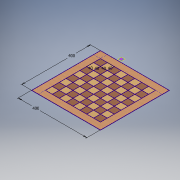
# Autodesk Inventor part: Lid
Saved by Autodesk Inventor 2019 (Build 230136000, 136)
## iProperties
Created: 2019-08-21
Part Number: Lid
Material: Generic
Document SubType Name: Modeling
Designer: Bruno
Density: 1 g/cm^3
Appearance: Default
Author: Bruno
Autodesk Inventor part; units mm, degrees
ref_plane "YZ Plane" through (0, 0, 0) normal (1, 0, 0) x (0, 1, 0)
ref_plane "XZ Plane" through (0, 0, 0) normal (0, 1, 0) x (-1, 0, 0)
ref_plane "XY Plane" through (0, 0, 0) normal (0, 0, 1) x (1, 0, 0)
ref_plane "Work Plane4" through (0, -2, 0) normal (0, -1, 0) x (1, 0, 0)
sketch "Sketch2" plane through (0, -2, 0) normal (0, -1, 0) x (1, 0, 0)
  line L0 (-64.9312, 57.9049) -> (-24.9312, 57.9049)
  line L1 (-24.9312, 57.9049) -> (-24.9312, 97.9049)
  line L2 (-24.9312, 97.9049) -> (-64.9312, 97.9049)
  line L3 (-64.9312, 97.9049) -> (-64.9312, 57.9049)
  line L4 (-24.9312, 137.9049) -> (-64.9312, 137.9049)
  line L5 (-24.9312, 97.9049) -> (-24.9312, 137.9049)
  line L6 (-64.9312, 97.9049) -> (-24.9312, 97.9049)
  line L7 (-64.9312, 137.9049) -> (-64.9312, 97.9049)
  line L8 (-24.9312, 177.9049) -> (-64.9312, 177.9049)
  line L9 (-24.9312, 137.9049) -> (-24.9312, 177.9049)
  line L10 (-64.9312, 137.9049) -> (-24.9312, 137.9049)
  line L11 (-64.9312, 177.9049) -> (-64.9312, 137.9049)
  line L12 (-24.9312, 217.9049) -> (-64.9312, 217.9049)
  line L13 (-24.9312, 177.9049) -> (-24.9312, 217.9049)
  line L14 (-64.9312, 177.9049) -> (-24.9312, 177.9049)
  line L15 (-64.9312, 217.9049) -> (-64.9312, 177.9049)
  line L16 (-24.9312, 257.9049) -> (-64.9312, 257.9049)
  line L17 (-24.9312, 217.9049) -> (-24.9312, 257.9049)
  line L18 (-64.9312, 217.9049) -> (-24.9312, 217.9049)
  line L19 (-64.9312, 257.9049) -> (-64.9312, 217.9049)
  line L20 (-24.9312, 297.9049) -> (-64.9312, 297.9049)
  line L21 (-24.9312, 257.9049) -> (-24.9312, 297.9049)
  line L22 (-64.9312, 257.9049) -> (-24.9312, 257.9049)
  line L23 (-64.9312, 297.9049) -> (-64.9312, 257.9049)
  line L24 (-24.9312, 337.9049) -> (-64.9312, 337.9049)
  line L25 (-24.9312, 297.9049) -> (-24.9312, 337.9049)
  line L26 (-64.9312, 297.9049) -> (-24.9312, 297.9049)
  line L27 (-64.9312, 337.9049) -> (-64.9312, 297.9049)
  line L28 (-24.9312, 377.9049) -> (-64.9312, 377.9049)
  line L29 (-24.9312, 337.9049) -> (-24.9312, 377.9049)
  line L30 (-64.9312, 337.9049) -> (-24.9312, 337.9049)
  line L31 (-64.9312, 377.9049) -> (-64.9312, 337.9049)
  line L32 (15.0688, 97.9049) -> (-24.9312, 97.9049)
  line L33 (15.0688, 57.9049) -> (15.0688, 97.9049)
  line L34 (-24.9312, 57.9049) -> (15.0688, 57.9049)
  line L35 (-24.9312, 97.9049) -> (-24.9312, 57.9049)
  line L36 (15.0688, 137.9049) -> (-24.9312, 137.9049)
  line L37 (15.0688, 97.9049) -> (15.0688, 137.9049)
  line L38 (-24.9312, 97.9049) -> (15.0688, 97.9049)
  line L39 (-24.9312, 137.9049) -> (-24.9312, 97.9049)
  line L40 (15.0688, 177.9049) -> (-24.9312, 177.9049)
  line L41 (15.0688, 137.9049) -> (15.0688, 177.9049)
  line L42 (-24.9312, 137.9049) -> (15.0688, 137.9049)
  line L43 (-24.9312, 177.9049) -> (-24.9312, 137.9049)
  line L44 (15.0688, 217.9049) -> (-24.9312, 217.9049)
  line L45 (15.0688, 177.9049) -> (15.0688, 217.9049)
  line L46 (-24.9312, 177.9049) -> (15.0688, 177.9049)
  line L47 (-24.9312, 217.9049) -> (-24.9312, 177.9049)
  line L48 (15.0688, 257.9049) -> (-24.9312, 257.9049)
  line L49 (15.0688, 217.9049) -> (15.0688, 257.9049)
  line L50 (-24.9312, 217.9049) -> (15.0688, 217.9049)
  line L51 (-24.9312, 257.9049) -> (-24.9312, 217.9049)
  line L52 (15.0688, 297.9049) -> (-24.9312, 297.9049)
  line L53 (15.0688, 257.9049) -> (15.0688, 297.9049)
  line L54 (-24.9312, 257.9049) -> (15.0688, 257.9049)
  line L55 (-24.9312, 297.9049) -> (-24.9312, 257.9049)
  line L56 (15.0688, 337.9049) -> (-24.9312, 337.9049)
  line L57 (15.0688, 297.9049) -> (15.0688, 337.9049)
  line L58 (-24.9312, 297.9049) -> (15.0688, 297.9049)
  line L59 (-24.9312, 337.9049) -> (-24.9312, 297.9049)
  line L60 (15.0688, 377.9049) -> (-24.9312, 377.9049)
  line L61 (15.0688, 337.9049) -> (15.0688, 377.9049)
  line L62 (-24.9312, 337.9049) -> (15.0688, 337.9049)
  line L63 (-24.9312, 377.9049) -> (-24.9312, 337.9049)
  line L64 (55.0688, 97.9049) -> (15.0688, 97.9049)
  line L65 (55.0688, 57.9049) -> (55.0688, 97.9049)
  line L66 (15.0688, 57.9049) -> (55.0688, 57.9049)
  line L67 (15.0688, 97.9049) -> (15.0688, 57.9049)
  line L68 (55.0688, 137.9049) -> (15.0688, 137.9049)
  line L69 (55.0688, 97.9049) -> (55.0688, 137.9049)
  line L70 (15.0688, 97.9049) -> (55.0688, 97.9049)
  line L71 (15.0688, 137.9049) -> (15.0688, 97.9049)
  line L72 (55.0688, 177.9049) -> (15.0688, 177.9049)
  line L73 (55.0688, 137.9049) -> (55.0688, 177.9049)
  line L74 (15.0688, 137.9049) -> (55.0688, 137.9049)
  line L75 (15.0688, 177.9049) -> (15.0688, 137.9049)
  line L76 (55.0688, 217.9049) -> (15.0688, 217.9049)
  line L77 (55.0688, 177.9049) -> (55.0688, 217.9049)
  line L78 (15.0688, 177.9049) -> (55.0688, 177.9049)
  line L79 (15.0688, 217.9049) -> (15.0688, 177.9049)
  line L80 (55.0688, 257.9049) -> (15.0688, 257.9049)
  line L81 (55.0688, 217.9049) -> (55.0688, 257.9049)
  line L82 (15.0688, 217.9049) -> (55.0688, 217.9049)
  line L83 (15.0688, 257.9049) -> (15.0688, 217.9049)
  line L84 (55.0688, 297.9049) -> (15.0688, 297.9049)
  line L85 (55.0688, 257.9049) -> (55.0688, 297.9049)
  line L86 (15.0688, 257.9049) -> (55.0688, 257.9049)
  line L87 (15.0688, 297.9049) -> (15.0688, 257.9049)
  line L88 (55.0688, 337.9049) -> (15.0688, 337.9049)
  line L89 (55.0688, 297.9049) -> (55.0688, 337.9049)
  line L90 (15.0688, 297.9049) -> (55.0688, 297.9049)
  line L91 (15.0688, 337.9049) -> (15.0688, 297.9049)
  line L92 (55.0688, 377.9049) -> (15.0688, 377.9049)
  line L93 (55.0688, 337.9049) -> (55.0688, 377.9049)
  line L94 (15.0688, 337.9049) -> (55.0688, 337.9049)
  line L95 (15.0688, 377.9049) -> (15.0688, 337.9049)
  line L96 (95.0688, 97.9049) -> (55.0688, 97.9049)
  line L97 (95.0688, 57.9049) -> (95.0688, 97.9049)
  line L98 (55.0688, 57.9049) -> (95.0688, 57.9049)
  line L99 (55.0688, 97.9049) -> (55.0688, 57.9049)
  line L100 (95.0688, 137.9049) -> (55.0688, 137.9049)
  line L101 (95.0688, 97.9049) -> (95.0688, 137.9049)
  line L102 (55.0688, 97.9049) -> (95.0688, 97.9049)
  line L103 (55.0688, 137.9049) -> (55.0688, 97.9049)
  line L104 (95.0688, 177.9049) -> (55.0688, 177.9049)
  line L105 (95.0688, 137.9049) -> (95.0688, 177.9049)
  line L106 (55.0688, 137.9049) -> (95.0688, 137.9049)
  line L107 (55.0688, 177.9049) -> (55.0688, 137.9049)
  line L108 (95.0688, 217.9049) -> (55.0688, 217.9049)
  line L109 (95.0688, 177.9049) -> (95.0688, 217.9049)
  line L110 (55.0688, 177.9049) -> (95.0688, 177.9049)
  line L111 (55.0688, 217.9049) -> (55.0688, 177.9049)
  line L112 (95.0688, 257.9049) -> (55.0688, 257.9049)
  line L113 (95.0688, 217.9049) -> (95.0688, 257.9049)
  line L114 (55.0688, 217.9049) -> (95.0688, 217.9049)
  line L115 (55.0688, 257.9049) -> (55.0688, 217.9049)
  line L116 (95.0688, 297.9049) -> (55.0688, 297.9049)
  line L117 (95.0688, 257.9049) -> (95.0688, 297.9049)
  line L118 (55.0688, 257.9049) -> (95.0688, 257.9049)
  line L119 (55.0688, 297.9049) -> (55.0688, 257.9049)
  line L120 (95.0688, 337.9049) -> (55.0688, 337.9049)
  line L121 (95.0688, 297.9049) -> (95.0688, 337.9049)
  line L122 (55.0688, 297.9049) -> (95.0688, 297.9049)
  line L123 (55.0688, 337.9049) -> (55.0688, 297.9049)
  line L124 (95.0688, 377.9049) -> (55.0688, 377.9049)
  line L125 (95.0688, 337.9049) -> (95.0688, 377.9049)
  line L126 (55.0688, 337.9049) -> (95.0688, 337.9049)
  line L127 (55.0688, 377.9049) -> (55.0688, 337.9049)
  line L128 (135.0688, 97.9049) -> (95.0688, 97.9049)
  line L129 (135.0688, 57.9049) -> (135.0688, 97.9049)
  line L130 (95.0688, 57.9049) -> (135.0688, 57.9049)
  line L131 (95.0688, 97.9049) -> (95.0688, 57.9049)
  line L132 (135.0688, 137.9049) -> (95.0688, 137.9049)
  line L133 (135.0688, 97.9049) -> (135.0688, 137.9049)
  line L134 (95.0688, 97.9049) -> (135.0688, 97.9049)
  line L135 (95.0688, 137.9049) -> (95.0688, 97.9049)
  line L136 (135.0688, 177.9049) -> (95.0688, 177.9049)
  line L137 (135.0688, 137.9049) -> (135.0688, 177.9049)
  line L138 (95.0688, 137.9049) -> (135.0688, 137.9049)
  line L139 (95.0688, 177.9049) -> (95.0688, 137.9049)
  line L140 (135.0688, 217.9049) -> (95.0688, 217.9049)
  line L141 (135.0688, 177.9049) -> (135.0688, 217.9049)
  line L142 (95.0688, 177.9049) -> (135.0688, 177.9049)
  line L143 (95.0688, 217.9049) -> (95.0688, 177.9049)
  line L144 (135.0688, 257.9049) -> (95.0688, 257.9049)
  line L145 (135.0688, 217.9049) -> (135.0688, 257.9049)
  line L146 (95.0688, 217.9049) -> (135.0688, 217.9049)
  line L147 (95.0688, 257.9049) -> (95.0688, 217.9049)
  line L148 (135.0688, 297.9049) -> (95.0688, 297.9049)
  line L149 (135.0688, 257.9049) -> (135.0688, 297.9049)
  line L150 (95.0688, 257.9049) -> (135.0688, 257.9049)
  line L151 (95.0688, 297.9049) -> (95.0688, 257.9049)
  line L152 (135.0688, 337.9049) -> (95.0688, 337.9049)
  line L153 (135.0688, 297.9049) -> (135.0688, 337.9049)
  line L154 (95.0688, 297.9049) -> (135.0688, 297.9049)
  line L155 (95.0688, 337.9049) -> (95.0688, 297.9049)
  line L156 (135.0688, 377.9049) -> (95.0688, 377.9049)
  line L157 (135.0688, 337.9049) -> (135.0688, 377.9049)
  line L158 (95.0688, 337.9049) -> (135.0688, 337.9049)
  line L159 (95.0688, 377.9049) -> (95.0688, 337.9049)
  line L160 (175.0688, 97.9049) -> (135.0688, 97.9049)
  line L161 (175.0688, 57.9049) -> (175.0688, 97.9049)
  line L162 (135.0688, 57.9049) -> (175.0688, 57.9049)
  line L163 (135.0688, 97.9049) -> (135.0688, 57.9049)
  line L164 (175.0688, 137.9049) -> (135.0688, 137.9049)
  line L165 (175.0688, 97.9049) -> (175.0688, 137.9049)
  line L166 (135.0688, 97.9049) -> (175.0688, 97.9049)
  line L167 (135.0688, 137.9049) -> (135.0688, 97.9049)
  line L168 (175.0688, 177.9049) -> (135.0688, 177.9049)
  line L169 (175.0688, 137.9049) -> (175.0688, 177.9049)
  line L170 (135.0688, 137.9049) -> (175.0688, 137.9049)
  line L171 (135.0688, 177.9049) -> (135.0688, 137.9049)
  line L172 (175.0688, 217.9049) -> (135.0688, 217.9049)
  line L173 (175.0688, 177.9049) -> (175.0688, 217.9049)
  line L174 (135.0688, 177.9049) -> (175.0688, 177.9049)
  line L175 (135.0688, 217.9049) -> (135.0688, 177.9049)
  line L176 (175.0688, 257.9049) -> (135.0688, 257.9049)
  line L177 (175.0688, 217.9049) -> (175.0688, 257.9049)
  line L178 (135.0688, 217.9049) -> (175.0688, 217.9049)
  line L179 (135.0688, 257.9049) -> (135.0688, 217.9049)
  line L180 (175.0688, 297.9049) -> (135.0688, 297.9049)
  line L181 (175.0688, 257.9049) -> (175.0688, 297.9049)
  line L182 (135.0688, 257.9049) -> (175.0688, 257.9049)
  line L183 (135.0688, 297.9049) -> (135.0688, 257.9049)
  line L184 (175.0688, 337.9049) -> (135.0688, 337.9049)
  line L185 (175.0688, 297.9049) -> (175.0688, 337.9049)
  line L186 (135.0688, 297.9049) -> (175.0688, 297.9049)
  line L187 (135.0688, 337.9049) -> (135.0688, 297.9049)
  line L188 (175.0688, 377.9049) -> (135.0688, 377.9049)
  line L189 (175.0688, 337.9049) -> (175.0688, 377.9049)
  line L190 (135.0688, 337.9049) -> (175.0688, 337.9049)
  line L191 (135.0688, 377.9049) -> (135.0688, 337.9049)
  line L192 (215.0688, 97.9049) -> (175.0688, 97.9049)
  line L193 (215.0688, 57.9049) -> (215.0688, 97.9049)
  line L194 (175.0688, 57.9049) -> (215.0688, 57.9049)
  line L195 (175.0688, 97.9049) -> (175.0688, 57.9049)
  line L196 (215.0688, 137.9049) -> (175.0688, 137.9049)
  line L197 (215.0688, 97.9049) -> (215.0688, 137.9049)
  line L198 (175.0688, 97.9049) -> (215.0688, 97.9049)
  line L199 (175.0688, 137.9049) -> (175.0688, 97.9049)
  line L200 (215.0688, 177.9049) -> (175.0688, 177.9049)
  line L201 (215.0688, 137.9049) -> (215.0688, 177.9049)
  line L202 (175.0688, 137.9049) -> (215.0688, 137.9049)
  line L203 (175.0688, 177.9049) -> (175.0688, 137.9049)
  line L204 (215.0688, 217.9049) -> (175.0688, 217.9049)
  line L205 (215.0688, 177.9049) -> (215.0688, 217.9049)
  line L206 (175.0688, 177.9049) -> (215.0688, 177.9049)
  line L207 (175.0688, 217.9049) -> (175.0688, 177.9049)
  line L208 (215.0688, 257.9049) -> (175.0688, 257.9049)
  line L209 (215.0688, 217.9049) -> (215.0688, 257.9049)
  line L210 (175.0688, 217.9049) -> (215.0688, 217.9049)
  line L211 (175.0688, 257.9049) -> (175.0688, 217.9049)
  line L212 (215.0688, 297.9049) -> (175.0688, 297.9049)
  line L213 (215.0688, 257.9049) -> (215.0688, 297.9049)
  line L214 (175.0688, 257.9049) -> (215.0688, 257.9049)
  line L215 (175.0688, 297.9049) -> (175.0688, 257.9049)
  line L216 (215.0688, 337.9049) -> (175.0688, 337.9049)
  line L217 (215.0688, 297.9049) -> (215.0688, 337.9049)
  line L218 (175.0688, 297.9049) -> (215.0688, 297.9049)
  line L219 (175.0688, 337.9049) -> (175.0688, 297.9049)
  line L220 (215.0688, 377.9049) -> (175.0688, 377.9049)
  line L221 (215.0688, 337.9049) -> (215.0688, 377.9049)
  line L222 (175.0688, 337.9049) -> (215.0688, 337.9049)
  line L223 (175.0688, 377.9049) -> (175.0688, 337.9049)
  line L224 (255.0688, 97.9049) -> (215.0688, 97.9049)
  line L225 (255.0688, 57.9049) -> (255.0688, 97.9049)
  line L226 (215.0688, 57.9049) -> (255.0688, 57.9049)
  line L227 (215.0688, 97.9049) -> (215.0688, 57.9049)
  line L228 (255.0688, 137.9049) -> (215.0688, 137.9049)
  line L229 (255.0688, 97.9049) -> (255.0688, 137.9049)
  line L230 (215.0688, 97.9049) -> (255.0688, 97.9049)
  line L231 (215.0688, 137.9049) -> (215.0688, 97.9049)
  line L232 (255.0688, 177.9049) -> (215.0688, 177.9049)
  line L233 (255.0688, 137.9049) -> (255.0688, 177.9049)
  line L234 (215.0688, 137.9049) -> (255.0688, 137.9049)
  line L235 (215.0688, 177.9049) -> (215.0688, 137.9049)
  line L236 (255.0688, 217.9049) -> (215.0688, 217.9049)
  line L237 (255.0688, 177.9049) -> (255.0688, 217.9049)
  line L238 (215.0688, 177.9049) -> (255.0688, 177.9049)
  line L239 (215.0688, 217.9049) -> (215.0688, 177.9049)
  line L240 (255.0688, 257.9049) -> (215.0688, 257.9049)
  line L241 (255.0688, 217.9049) -> (255.0688, 257.9049)
  line L242 (215.0688, 217.9049) -> (255.0688, 217.9049)
  line L243 (215.0688, 257.9049) -> (215.0688, 217.9049)
  line L244 (255.0688, 297.9049) -> (215.0688, 297.9049)
  line L245 (255.0688, 257.9049) -> (255.0688, 297.9049)
  line L246 (215.0688, 257.9049) -> (255.0688, 257.9049)
  line L247 (215.0688, 297.9049) -> (215.0688, 257.9049)
  line L248 (255.0688, 337.9049) -> (215.0688, 337.9049)
  line L249 (255.0688, 297.9049) -> (255.0688, 337.9049)
  line L250 (215.0688, 297.9049) -> (255.0688, 297.9049)
  line L251 (215.0688, 337.9049) -> (215.0688, 297.9049)
  line L252 (255.0688, 377.9049) -> (215.0688, 377.9049)
  line L253 (255.0688, 337.9049) -> (255.0688, 377.9049)
  line L254 (215.0688, 337.9049) -> (255.0688, 337.9049)
  line L255 (215.0688, 377.9049) -> (215.0688, 337.9049)
  line L256 (-104.9312, 17.9049) -> (-104.9312, 417.9049)
  line L257 (-104.9312, 417.9049) -> (295.0688, 417.9049)
  line L258 (295.0688, 417.9049) -> (295.0688, 17.9049)
  line L259 (295.0688, 17.9049) -> (-104.9312, 17.9049)
  line L260 (-64.9312, 377.9049) -> (-64.9312, 417.9049) construction
  line L261 (-64.9312, 57.9049) -> (-64.9312, 17.9049) construction
  line L262 (-64.9312, 57.9049) -> (-104.9312, 57.9049) construction
  line L263 (255.0688, 57.9049) -> (295.0688, 57.9049) construction
  point P0 (0, 0)
  dimension "d4" = 40
  dimension "d5" = 40
  dimension "d8" = 40
  dimension "d11" = 40
  dimension "d14" = 400
  dimension "d15" = 400
  constraints: 528 end point, 7 perpendicular, 4 collinear, 4 point on line, 4 vertical, 3 horizontal, 2 parallel, 502 other
  measures "d4" distance of L2.end L1.end
  measures "d5" distance of L1.end L0.end
  measures "d8" distance of L1.end L4.start
  measures "d11" distance of L1.end L32.start
  measures "d14" distance of L256.end L257.end
  measures "d15" distance of L256.start L256.end
extrude "Extrusion2" add sketch "Sketch2" along normal blind 2
extrude "Extrusion3" add sketch "Sketch2" along normal blind 2 separate body contours L1 L32 L33 L34 | L7 L4 L5 L2 | L9 L40 L41 L36 | L37 L68 L69 L64 | L65 L96 L97 L98 | L15 L12 L13 L8 | L17 L48 L49 L44 | L45 L76 L77 L72 | L73 L104 L105 L100 | L101 L132 L133 L128 | L129 L160 L161 L162 | L23 L20 L21 L16 | L25 L56 L57 L52 | L53 L84 L85 L80 | L81 L112 L113 L108 | L109 L140 L141 L136 | L137 L168 L169 L164 | L165 L196 L197 L192 | L193 L224 L225 L226 | L31 L28 L29 L24 | L61 L92 L93 L88 | L89 L120 L121 L116 | L117 L148 L149 L144 | L145 L176 L177 L172 | L173 L204 L205 L200 | L201 L232 L233 L228 | L125 L156 L157 L152 | L153 L184 L185 L180 | L181 L212 L213 L208 | L209 L240 L241 L236 | L189 L220 L221 L216 | L217 L248 L249 L244
extrude "Extrusion4" add sketch "Sketch2" along normal blind 2 separate body contours L3 L2 L1 L0 | L5 L36 L37 L32 | L33 L64 L65 L66 | L11 L8 L9 L4 | L13 L44 L45 L40 | L41 L72 L73 L68 | L69 L100 L101 L96 | L97 L128 L129 L130 | L19 L16 L17 L12 | L21 L52 L53 L48 | L49 L80 L81 L76 | L77 L108 L109 L104 | L105 L136 L137 L132 | L133 L164 L165 L160 | L161 L192 L193 L194 | L27 L24 L25 L20 | L29 L60 L61 L56 | L57 L88 L89 L84 | L85 L116 L117 L112 | L113 L144 L145 L140 | L141 L172 L173 L168 | L169 L200 L201 L196 | L197 L228 L229 L224 | L93 L124 L125 L120 | L121 L152 L153 L148 | L149 L180 L181 L176 | L177 L208 L209 L204 | L205 L236 L237 L232 | L157 L188 L189 L184 | L185 L216 L217 L212 | L213 L244 L245 L240 | L221 L252 L253 L248
body "Solid2"
body "Solid3"
body "Solid4"
